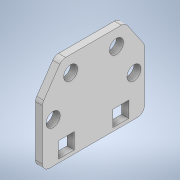
# Autodesk Inventor part: Практика галактика
Saved by Autodesk Inventor 2022 (Build 260153000, 153)
## iProperties
Created: 2022-07-09
Part Number: Практика галактика
Material: Типовые
Document SubType Name: Modeling
Designer: Константин
Density: 1 g/cm^3
Appearance: По умолчанию
Author: Константин
Autodesk Inventor part; units mm, degrees
ref_plane "YZ Plane" through (0, 0, 0) normal (1, 0, 0) x (0, 1, 0)
ref_plane "XZ Plane" through (0, 0, 0) normal (0, 1, 0) x (-1, 0, 0)
ref_plane "XY Plane" through (0, 0, 0) normal (0, 0, 1) x (1, 0, 0)
sketch "Эскиз1" plane through (0, 0, 0) normal (1, 0, 0) x (0, 1, 0)
  line L0 (152.4218, -265.1334) -> (152.4218, -277.6334)
  line L1 (152.4218, -277.6334) -> (177.4218, -277.6334)
  line L2 (177.4218, -277.6334) -> (177.4218, -269.6855)
  line L3 (176.5549, -268.0374) -> (169.9337, -263.4853)
  line L4 (154.4218, -263.1334) -> (168.8006, -263.1334)
  line L5 (153.4218, -267.6334) -> (157.9218, -267.6334)
  line L6 (157.9218, -267.6334) -> (157.9218, -272.1334)
  line L7 (157.9218, -272.1334) -> (153.4218, -272.1334)
  line L8 (153.4218, -272.1334) -> (153.4218, -267.6334)
  line L9 (177.4218, -277.6334) -> (177.4218, -269.6855)
  line L10 (176.5549, -268.0374) -> (169.9337, -263.4853)
  circle A0 centre (163.9218, -266.1334) radius 2
  circle A1 centre (172.9218, -271.1334) radius 2
  arc A2 (154.4218, -263.1334) -> (152.4218, -265.1334) centre (154.4218, -265.1334) ccw
  arc A3 (169.9337, -263.4853) -> (168.8006, -263.1334) centre (168.8006, -265.1334) ccw
  arc A4 (177.4218, -269.6855) -> (176.5549, -268.0374) centre (175.4218, -269.6855) ccw
  line L11 (152.4218, -290.1334) -> (152.4218, -277.6334)
  line L12 (177.4218, -277.6334) -> (177.4218, -285.5814)
  line L13 (176.5549, -287.2295) -> (169.9337, -291.7815)
  circle A5 centre (172.9218, -284.1334) radius 2
  circle A6 centre (163.9218, -289.1334) radius 2
  line L14 (157.9218, -287.6334) -> (157.9218, -283.1334)
  line L15 (157.9218, -283.1334) -> (153.4218, -283.1334)
  line L16 (153.4218, -283.1334) -> (153.4218, -287.6334)
  line L17 (154.4218, -292.1334) -> (168.8006, -292.1334)
  line L18 (153.4218, -287.6334) -> (157.9218, -287.6334)
  arc A7 (152.4218, -290.1334) -> (154.4218, -292.1334) centre (154.4218, -290.1334) ccw
  arc A8 (168.8006, -292.1334) -> (169.9337, -291.7815) centre (168.8006, -290.1334) ccw
  arc A9 (176.5549, -287.2295) -> (177.4218, -285.5814) centre (175.4218, -285.5814) ccw
  dimension "d181" = 5.5
  dimension "d182" = 1
  dimension "d183" = 4.5
  dimension "d184" = 4.5
  dimension "d185" = 6
  dimension "d186" = 5
  dimension "d187" = 3
  dimension "d188" = 9
  constraints: 38 end point, 15 symmetric about line, 12 point on circle, 10 centre point, 5 tangent, 2 equal radius, 2 vertical, 1 horizontal, 5 other
  measures "d181" distance between parallel lines of L1 L7
  measures "d182" distance between parallel lines of L0 L8
  measures "d183" distance of L6.end L7.end
  measures "d184" distance of L6.start L6.end
  measures "d185" distance from line of L6 A0.centre
  measures "d186" vertical distance of A0.centre A1.centre
  measures "d187" distance from line of L4 A0.centre
  measures "d188" horizontal distance of A0.centre A1.centre
extrude "Выдавливание3" add sketch "Эскиз1" along normal blind 2
